Autodesk Fusion 360 part; units mm, degrees
(part 2 of 6)
sketch "Cell axial cylinder sketch (2)" plane through (0, 9.2, 0) normal (0, 1, 0) x (1, 0, 0) in component "Battery / 18650 cell B - owner-rated 3400 mAh"
  circle A0 centre (34.2, -26.95) radius 9.1
  dimension "d462" = 34.2
  dimension "d463" = 26.95
  dimension "d464" = 9.1
  measures "d462" horizontal distance of origin A0.centre
  measures "d463" vertical distance of origin A0.centre
  measures "d464" radius of A0
extrude "Blue 18650 reference cylinder'" add sketch "Cell axial cylinder sketch (2)" along normal blind 69 separate body makes body 19 in component "Battery / 18650 cell B - owner-rated 3400 mAh"
ref_plane "WorkPlane1" through (0, 0, 43) normal (0, 0, 1) x (1, 0, 0) in component "Battery / red RCY disconnect body - provisional reference"
sketch "Red battery disconnect reference body sketch" plane through (0, 0, 43) normal (0, 0, 1) x (1, 0, 0) in component "Battery / red RCY disconnect body - provisional reference"
  line L0 (29, 70) -> (41, 70)
  line L1 (41, 70) -> (41, 80)
  line L2 (41, 80) -> (29, 80)
  line L3 (29, 80) -> (29, 70)
  dimension "d469" = 29
  dimension "d470" = 70
  dimension "d471" = 12
  dimension "d472" = 10
  constraint horizontal L0
  constraint vertical L1
  constraint horizontal L2
  constraint vertical L3
  measures "d469" horizontal distance of origin L0.start
  measures "d470" vertical distance of origin L0.start
  measures "d471" horizontal distance of L0.start L0.end
  measures "d472" vertical distance of L0.end L1.end
extrude "Red battery disconnect reference body" add sketch "Red battery disconnect reference body sketch" along normal blind 4 separate body makes body 20 in component "Battery / red RCY disconnect body - provisional reference"
ref_plane "WorkPlane2" through (0, 0, 42.9) normal (0, 0, 1) x (1, 0, 0) in component "Battery / red RCY disconnect body - provisional reference"
sketch "Illustrative disconnect key groove sketch" plane through (0, 0, 42.9) normal (0, 0, 1) x (1, 0, 0) in component "Battery / red RCY disconnect body - provisional reference"
  line L0 (34.4, 69.9) -> (35.6, 69.9)
  line L1 (35.6, 69.9) -> (35.6, 80.1)
  line L2 (35.6, 80.1) -> (34.4, 80.1)
  line L3 (34.4, 80.1) -> (34.4, 69.9)
  dimension "d477" = 34.4
  dimension "d478" = 69.9
  dimension "d479" = 1.2
  dimension "d480" = 10.2
  constraint horizontal L0
  constraint vertical L1
  constraint horizontal L2
  constraint vertical L3
  measures "d477" horizontal distance of origin L0.start
  measures "d478" vertical distance of origin L0.start
  measures "d479" horizontal distance of L0.start L0.end
  measures "d480" vertical distance of L0.end L1.end
extrude "Illustrative disconnect key groove" cut sketch "Illustrative disconnect key groove sketch" along normal blind 0.7 bodies 20 in component "Battery / red RCY disconnect body - provisional reference"
ref_plane "WorkPlane1" through (0, 0, 47) normal (0, 0, 1) x (1, 0, 0) in component "Battery / red RCY disconnect mate - provisional reference"
sketch "Red battery disconnect mating reference sketch" plane through (0, 0, 47) normal (0, 0, 1) x (1, 0, 0) in component "Battery / red RCY disconnect mate - provisional reference"
  line L0 (29, 70) -> (41, 70)
  line L1 (41, 70) -> (41, 80)
  line L2 (41, 80) -> (29, 80)
  line L3 (29, 80) -> (29, 70)
  dimension "d485" = 29
  dimension "d486" = 70
  dimension "d487" = 12
  dimension "d488" = 10
  constraint horizontal L0
  constraint vertical L1
  constraint horizontal L2
  constraint vertical L3
  measures "d485" horizontal distance of origin L0.start
  measures "d486" vertical distance of origin L0.start
  measures "d487" horizontal distance of L0.start L0.end
  measures "d488" vertical distance of L0.end L1.end
extrude "Red battery disconnect mating reference" add sketch "Red battery disconnect mating reference sketch" along normal blind 2.2 separate body makes body 21 in component "Battery / red RCY disconnect mate - provisional reference"
ref_plane "WorkPlane16" through (0, 0, 37.65) normal (0, 0, 1) x (1, 0, 0) in component "01 Tapered printed housing"
sketch "Carrier bottom wall bracket sketch" plane through (0, 0, 37.65) normal (0, 0, 1) x (1, 0, 0) in component "01 Tapered printed housing"
  line L0 (36.2, 2.1) -> (43.8, 2.1)
  line L1 (43.8, 2.1) -> (43.8, 14.1)
  line L2 (43.8, 14.1) -> (36.2, 14.1)
  line L3 (36.2, 14.1) -> (36.2, 2.1)
  dimension "d493" = 36.2
  dimension "d494" = 2.1
  dimension "d495" = 7.6
  dimension "d496" = 12
  constraint horizontal L0
  constraint vertical L1
  constraint horizontal L2
  constraint vertical L3
  measures "d493" horizontal distance of origin L0.start
  measures "d494" vertical distance of origin L0.start
  measures "d495" horizontal distance of L0.start L0.end
  measures "d496" vertical distance of L0.end L1.end
extrude "Carrier bottom wall bracket" add sketch "Carrier bottom wall bracket sketch" along normal blind 6 bodies 1 in component "01 Tapered printed housing"
ref_plane "WorkPlane17" through (0, 0, 37.65) normal (0, 0, 1) x (1, 0, 0) in component "01 Tapered printed housing"
sketch "Carrier M2 boss sketch" plane through (0, 0, 37.65) normal (0, 0, 1) x (1, 0, 0) in component "01 Tapered printed housing"
  circle A0 centre (6, 18) radius 3.8
  dimension "d501" = 6
  dimension "d502" = 18
  dimension "d503" = 3.8
  measures "d501" horizontal distance of origin A0.centre
  measures "d502" vertical distance of origin A0.centre
  measures "d503" radius of A0
extrude "Carrier M2 boss" add sketch "Carrier M2 boss sketch" along normal blind 6 bodies 1 in component "01 Tapered printed housing"
ref_plane "WorkPlane18" through (0, 0, 39.65) normal (0, 0, 1) x (1, 0, 0) in component "01 Tapered printed housing"
sketch "Carrier insert pocket sketch" plane through (0, 0, 39.65) normal (0, 0, 1) x (1, 0, 0) in component "01 Tapered printed housing"
  circle A0 centre (6, 18) radius 1.65
  dimension "d508" = 6
  dimension "d509" = 18
  dimension "d510" = 1.65
  measures "d508" horizontal distance of origin A0.centre
  measures "d509" vertical distance of origin A0.centre
  measures "d510" radius of A0
extrude "Carrier insert pocket" cut sketch "Carrier insert pocket sketch" along normal blind 4.1 bodies 1 in component "01 Tapered printed housing"
ref_plane "WorkPlane19" through (0, 0, 37.65) normal (0, 0, 1) x (1, 0, 0) in component "01 Tapered printed housing"
sketch "Carrier M2 boss sketch (1)" plane through (0, 0, 37.65) normal (0, 0, 1) x (1, 0, 0) in component "01 Tapered printed housing"
  circle A0 centre (6, 77) radius 3.8
  dimension "d515" = 6
  dimension "d516" = 77
  dimension "d517" = 3.8
  measures "d515" horizontal distance of origin A0.centre
  measures "d516" vertical distance of origin A0.centre
  measures "d517" radius of A0
extrude "Carrier M2 boss (1)" add sketch "Carrier M2 boss sketch (1)" along normal blind 6 bodies 1 in component "01 Tapered printed housing"
ref_plane "WorkPlane20" through (0, 0, 39.65) normal (0, 0, 1) x (1, 0, 0) in component "01 Tapered printed housing"
sketch "Carrier insert pocket sketch (1)" plane through (0, 0, 39.65) normal (0, 0, 1) x (1, 0, 0) in component "01 Tapered printed housing"
  circle A0 centre (6, 77) radius 1.65
  dimension "d522" = 6
  dimension "d523" = 77
  dimension "d524" = 1.65
  measures "d522" horizontal distance of origin A0.centre
  measures "d523" vertical distance of origin A0.centre
  measures "d524" radius of A0
extrude "Carrier insert pocket (1)" cut sketch "Carrier insert pocket sketch (1)" along normal blind 4.1 bodies 1 in component "01 Tapered printed housing"
ref_plane "WorkPlane21" through (0, 0, 37.65) normal (0, 0, 1) x (1, 0, 0) in component "01 Tapered printed housing"
sketch "Carrier M2 boss sketch (2)" plane through (0, 0, 37.65) normal (0, 0, 1) x (1, 0, 0) in component "01 Tapered printed housing"
  circle A0 centre (40, 14) radius 3.8
  dimension "d529" = 40
  dimension "d530" = 14
  dimension "d531" = 3.8
  measures "d529" horizontal distance of origin A0.centre
  measures "d530" vertical distance of origin A0.centre
  measures "d531" radius of A0
extrude "Carrier M2 boss (2)" add sketch "Carrier M2 boss sketch (2)" along normal blind 6 bodies 1 in component "01 Tapered printed housing"
ref_plane "WorkPlane22" through (0, 0, 39.65) normal (0, 0, 1) x (1, 0, 0) in component "01 Tapered printed housing"
sketch "Carrier insert pocket sketch (2)" plane through (0, 0, 39.65) normal (0, 0, 1) x (1, 0, 0) in component "01 Tapered printed housing"
  circle A0 centre (40, 14) radius 1.65
  dimension "d536" = 40
  dimension "d537" = 14
  dimension "d538" = 1.65
  measures "d536" horizontal distance of origin A0.centre
  measures "d537" vertical distance of origin A0.centre
  measures "d538" radius of A0
extrude "Carrier insert pocket (2)" cut sketch "Carrier insert pocket sketch (2)" along normal blind 4.1 bodies 1 in component "01 Tapered printed housing"
ref_plane "WorkPlane1" through (0, 0, 43.65) normal (0, 0, 1) x (1, 0, 0) in component "Carrier / removable electronics plate"
sketch "Shaped electronics carrier sketch" plane through (0, 0, 43.65) normal (0, 0, 1) x (1, 0, 0) in component "Carrier / removable electronics plate"
  line L0 (2.7, 10.4) -> (43.6, 10.4)
  line L1 (43.6, 10.4) -> (43.6, 83.6)
  line L2 (43.6, 83.6) -> (2.7, 83.6)
  line L3 (2.7, 83.6) -> (2.7, 10.4)
  dimension "d543" = 2.7
  dimension "d544" = 10.4
  dimension "d545" = 40.9
  dimension "d546" = 73.2
  constraint horizontal L0
  constraint vertical L1
  constraint horizontal L2
  constraint vertical L3
  measures "d543" horizontal distance of origin L0.start
  measures "d544" vertical distance of origin L0.start
  measures "d545" horizontal distance of L0.start L0.end
  measures "d546" vertical distance of L0.end L1.end
extrude "Shaped electronics carrier" add sketch "Shaped electronics carrier sketch" along normal blind 2 separate body makes body 22 in component "Carrier / removable electronics plate"
ref_plane "WorkPlane1" through (0, 0, 45.65) normal (0, 0, 1) x (1, 0, 0) in component "Carrier / future PCB allocation — layout pending"
sketch "Reshaped future PCB sketch" plane through (0, 0, 45.65) normal (0, 0, 1) x (1, 0, 0) in component "Carrier / future PCB allocation — layout pending"
  line L0 (3.6, 12) -> (43, 12)
  line L1 (43, 12) -> (43, 82.4)
  line L2 (43, 82.4) -> (3.6, 82.4)
  line L3 (3.6, 82.4) -> (3.6, 12)
  dimension "d551" = 3.6
  dimension "d552" = 12
  dimension "d553" = 39.4
  dimension "d554" = 70.4
  constraint horizontal L0
  constraint vertical L1
  constraint horizontal L2
  constraint vertical L3
  measures "d551" horizontal distance of origin L0.start
  measures "d552" vertical distance of origin L0.start
  measures "d553" horizontal distance of L0.start L0.end
  measures "d554" vertical distance of L0.end L1.end
extrude "Reshaped future PCB" add sketch "Reshaped future PCB sketch" along normal blind 1.6 separate body makes body 23 in component "Carrier / future PCB allocation — layout pending"
ref_plane "WorkPlane2" through (0, 0, 43.5) normal (0, 0, 1) x (1, 0, 0) in component "Carrier / removable electronics plate"
sketch "Right button and terminal service notch sketch" plane through (0, 0, 43.5) normal (0, 0, 1) x (1, 0, 0) in component "Carrier / removable electronics plate"
  line L0 (2, 37) -> (26, 37)
  line L1 (26, 37) -> (26, 53)
  line L2 (26, 53) -> (2, 53)
  line L3 (2, 53) -> (2, 37)
  dimension "d559" = 2
  dimension "d560" = 37
  dimension "d561" = 24
  dimension "d562" = 16
  constraint horizontal L0
  constraint vertical L1
  constraint horizontal L2
  constraint vertical L3
  measures "d559" horizontal distance of origin L0.start
  measures "d560" vertical distance of origin L0.start
  measures "d561" horizontal distance of L0.start L0.end
  measures "d562" vertical distance of L0.end L1.end
extrude "Right button and terminal service notch" cut sketch "Right button and terminal service notch sketch" along normal blind 4 bodies 22 in component "Carrier / removable electronics plate"
ref_plane "WorkPlane3" through (0, 0, 43.5) normal (0, 0, 1) x (1, 0, 0) in component "Carrier / removable electronics plate"
sketch "Battery disconnect access notch sketch" plane through (0, 0, 43.5) normal (0, 0, 1) x (1, 0, 0) in component "Carrier / removable electronics plate"
  line L0 (28, 67) -> (44, 67)
  line L1 (44, 67) -> (44, 84)
  line L2 (44, 84) -> (28, 84)
  line L3 (28, 84) -> (28, 67)
  dimension "d567" = 28
  dimension "d568" = 67
  dimension "d569" = 16
  dimension "d570" = 17
  constraint horizontal L0
  constraint vertical L1
  constraint horizontal L2
  constraint vertical L3
  measures "d567" horizontal distance of origin L0.start
  measures "d568" vertical distance of origin L0.start
  measures "d569" horizontal distance of L0.start L0.end
  measures "d570" vertical distance of L0.end L1.end
extrude "Battery disconnect access notch" cut sketch "Battery disconnect access notch sketch" along normal blind 4 bodies 22 in component "Carrier / removable electronics plate"
ref_plane "WorkPlane4" through (0, 0, 43.5) normal (0, 0, 1) x (1, 0, 0) in component "Carrier / removable electronics plate"
sketch "Shared M2 mounting clearance sketch" plane through (0, 0, 43.5) normal (0, 0, 1) x (1, 0, 0) in component "Carrier / removable electronics plate"
  circle A0 centre (6, 18) radius 1.2
  dimension "d575" = 6
  dimension "d576" = 18
  dimension "d577" = 1.2
  measures "d575" horizontal distance of origin A0.centre
  measures "d576" vertical distance of origin A0.centre
  measures "d577" radius of A0
extrude "Shared M2 mounting clearance" cut sketch "Shared M2 mounting clearance sketch" along normal blind 4 bodies 22 in component "Carrier / removable electronics plate"
ref_plane "WorkPlane5" through (0, 0, 43.5) normal (0, 0, 1) x (1, 0, 0) in component "Carrier / removable electronics plate"
sketch "Shared M2 mounting clearance sketch (1)" plane through (0, 0, 43.5) normal (0, 0, 1) x (1, 0, 0) in component "Carrier / removable electronics plate"
  circle A0 centre (6, 77) radius 1.2
  dimension "d582" = 6
  dimension "d583" = 77
  dimension "d584" = 1.2
  measures "d582" horizontal distance of origin A0.centre
  measures "d583" vertical distance of origin A0.centre
  measures "d584" radius of A0
extrude "Shared M2 mounting clearance (1)" cut sketch "Shared M2 mounting clearance sketch (1)" along normal blind 4 bodies 22 in component "Carrier / removable electronics plate"
ref_plane "WorkPlane6" through (0, 0, 43.5) normal (0, 0, 1) x (1, 0, 0) in component "Carrier / removable electronics plate"
sketch "Shared M2 mounting clearance sketch (2)" plane through (0, 0, 43.5) normal (0, 0, 1) x (1, 0, 0) in component "Carrier / removable electronics plate"
  circle A0 centre (40, 14) radius 1.2
  dimension "d589" = 40
  dimension "d590" = 14
  dimension "d591" = 1.2
  measures "d589" horizontal distance of origin A0.centre
  measures "d590" vertical distance of origin A0.centre
  measures "d591" radius of A0
extrude "Shared M2 mounting clearance (2)" cut sketch "Shared M2 mounting clearance sketch (2)" along normal blind 4 bodies 22 in component "Carrier / removable electronics plate"
ref_plane "WorkPlane2" through (0, 0, 43.5) normal (0, 0, 1) x (1, 0, 0) in component "Carrier / future PCB allocation — layout pending"
sketch "Right button and terminal service notch sketch (2)" plane through (0, 0, 43.5) normal (0, 0, 1) x (1, 0, 0) in component "Carrier / future PCB allocation — layout pending"
  line L0 (2, 37) -> (26, 37)
  line L1 (26, 37) -> (26, 53)
  line L2 (26, 53) -> (2, 53)
  line L3 (2, 53) -> (2, 37)
  dimension "d596" = 2
  dimension "d597" = 37
  dimension "d598" = 24
  dimension "d599" = 16
  constraint horizontal L0
  constraint vertical L1
  constraint horizontal L2
  constraint vertical L3
  measures "d596" horizontal distance of origin L0.start
  measures "d597" vertical distance of origin L0.start
  measures "d598" horizontal distance of L0.start L0.end
  measures "d599" vertical distance of L0.end L1.end
extrude "Right button and terminal service notch'" cut sketch "Right button and terminal service notch sketch (2)" along normal blind 4 bodies 23 in component "Carrier / future PCB allocation — layout pending"
ref_plane "WorkPlane3" through (0, 0, 43.5) normal (0, 0, 1) x (1, 0, 0) in component "Carrier / future PCB allocation — layout pending"
sketch "Battery disconnect access notch sketch (2)" plane through (0, 0, 43.5) normal (0, 0, 1) x (1, 0, 0) in component "Carrier / future PCB allocation — layout pending"
  line L0 (28, 67) -> (44, 67)
  line L1 (44, 67) -> (44, 84)
  line L2 (44, 84) -> (28, 84)
  line L3 (28, 84) -> (28, 67)
  dimension "d604" = 28
  dimension "d605" = 67
  dimension "d606" = 16
  dimension "d607" = 17
  constraint horizontal L0
  constraint vertical L1
  constraint horizontal L2
  constraint vertical L3
  measures "d604" horizontal distance of origin L0.start
  measures "d605" vertical distance of origin L0.start
  measures "d606" horizontal distance of L0.start L0.end
  measures "d607" vertical distance of L0.end L1.end
extrude "Battery disconnect access notch'" cut sketch "Battery disconnect access notch sketch (2)" along normal blind 4 bodies 23 in component "Carrier / future PCB allocation — layout pending"
ref_plane "WorkPlane4" through (0, 0, 43.5) normal (0, 0, 1) x (1, 0, 0) in component "Carrier / future PCB allocation — layout pending"
sketch "Shared M2 mounting clearance sketch (3)" plane through (0, 0, 43.5) normal (0, 0, 1) x (1, 0, 0) in component "Carrier / future PCB allocation — layout pending"
  circle A0 centre (6, 18) radius 1.2
  dimension "d612" = 6
  dimension "d613" = 18
  dimension "d614" = 1.2
  measures "d612" horizontal distance of origin A0.centre
  measures "d613" vertical distance of origin A0.centre
  measures "d614" radius of A0
extrude "Shared M2 mounting clearance'" cut sketch "Shared M2 mounting clearance sketch (3)" along normal blind 4 bodies 23 in component "Carrier / future PCB allocation — layout pending"
ref_plane "WorkPlane5" through (0, 0, 43.5) normal (0, 0, 1) x (1, 0, 0) in component "Carrier / future PCB allocation — layout pending"
sketch "Shared M2 mounting clearance sketch (1) (2)" plane through (0, 0, 43.5) normal (0, 0, 1) x (1, 0, 0) in component "Carrier / future PCB allocation — layout pending"
  circle A0 centre (6, 77) radius 1.2
  dimension "d619" = 6
  dimension "d620" = 77
  dimension "d621" = 1.2
  measures "d619" horizontal distance of origin A0.centre
  measures "d620" vertical distance of origin A0.centre
  measures "d621" radius of A0
extrude "Shared M2 mounting clearance (1)'" cut sketch "Shared M2 mounting clearance sketch (1) (2)" along normal blind 4 bodies 23 in component "Carrier / future PCB allocation — layout pending"
ref_plane "WorkPlane6" through (0, 0, 43.5) normal (0, 0, 1) x (1, 0, 0) in component "Carrier / future PCB allocation — layout pending"
sketch "Shared M2 mounting clearance sketch (2) (2)" plane through (0, 0, 43.5) normal (0, 0, 1) x (1, 0, 0) in component "Carrier / future PCB allocation — layout pending"
  circle A0 centre (40, 14) radius 1.2
  dimension "d626" = 40
  dimension "d627" = 14
  dimension "d628" = 1.2
  measures "d626" horizontal distance of origin A0.centre
  measures "d627" vertical distance of origin A0.centre
  measures "d628" radius of A0
extrude "Shared M2 mounting clearance (2)'" cut sketch "Shared M2 mounting clearance sketch (2) (2)" along normal blind 4 bodies 23 in component "Carrier / future PCB allocation — layout pending"
ref_plane "WorkPlane7" through (0, 0, 47.25) normal (0, 0, 1) x (1, 0, 0) in component "Carrier / future PCB allocation — layout pending"
sketch "Power-stage allocation sketch" plane through (0, 0, 47.25) normal (0, 0, 1) x (1, 0, 0) in component "Carrier / future PCB allocation — layout pending"
  line L0 (12, 18) -> (32, 18)
  line L1 (32, 18) -> (32, 31)
  line L2 (32, 31) -> (12, 31)
  line L3 (12, 31) -> (12, 18)
  dimension "d633" = 12
  dimension "d634" = 18
  dimension "d635" = 20
  dimension "d636" = 13
  constraint horizontal L0
  constraint vertical L1
  constraint horizontal L2
  constraint vertical L3
  measures "d633" horizontal distance of origin L0.start
  measures "d634" vertical distance of origin L0.start
  measures "d635" horizontal distance of L0.start L0.end
  measures "d636" vertical distance of L0.end L1.end
extrude "Power-stage allocation" add sketch "Power-stage allocation sketch" along normal blind 3.5 separate body makes body 24 in component "Carrier / future PCB allocation — layout pending"
ref_plane "WorkPlane8" through (0, 0, 47.25) normal (0, 0, 1) x (1, 0, 0) in component "Carrier / future PCB allocation — layout pending"
sketch "Analog allocation sketch" plane through (0, 0, 47.25) normal (0, 0, 1) x (1, 0, 0) in component "Carrier / future PCB allocation — layout pending"
  line L0 (28, 40) -> (40, 40)
  line L1 (40, 40) -> (40, 59)
  line L2 (40, 59) -> (28, 59)
  line L3 (28, 59) -> (28, 40)
  dimension "d641" = 28
  dimension "d642" = 40
  dimension "d643" = 12
  dimension "d644" = 19
  constraint horizontal L0
  constraint vertical L1
  constraint horizontal L2
  constraint vertical L3
  measures "d641" horizontal distance of origin L0.start
  measures "d642" vertical distance of origin L0.start
  measures "d643" horizontal distance of L0.start L0.end
  measures "d644" vertical distance of L0.end L1.end
extrude "Analog allocation" add sketch "Analog allocation sketch" along normal blind 2.5 separate body makes body 25 in component "Carrier / future PCB allocation — layout pending"
ref_plane "WorkPlane9" through (0, 0, 47.25) normal (0, 0, 1) x (1, 0, 0) in component "Carrier / future PCB allocation — layout pending"
sketch "Digital allocation sketch" plane through (0, 0, 47.25) normal (0, 0, 1) x (1, 0, 0) in component "Carrier / future PCB allocation — layout pending"
  line L0 (12, 57) -> (24, 57)
  line L1 (24, 57) -> (24, 65)
  line L2 (24, 65) -> (12, 65)
  line L3 (12, 65) -> (12, 57)
  dimension "d649" = 12
  dimension "d650" = 57
  dimension "d651" = 12
  dimension "d652" = 8
  constraint horizontal L0
  constraint vertical L1
  constraint horizontal L2
  constraint vertical L3
  measures "d649" horizontal distance of origin L0.start
  measures "d650" vertical distance of origin L0.start
  measures "d651" horizontal distance of L0.start L0.end
  measures "d652" vertical distance of L0.end L1.end
extrude "Digital allocation" add sketch "Digital allocation sketch" along normal blind 2 separate body makes body 26 in component "Carrier / future PCB allocation — layout pending"
ref_plane "WorkPlane1" through (0, 0, -7) normal (0, 0, 1) x (1, 0, 0) in component "M2 x 7 socket_cap screw — GEN-M2-SHCS-L7-AF1.5"
sketch "Joined screw sketch (2)" plane through (0, 0, -7) normal (0, 0, 1) x (1, 0, 0) in component "M2 x 7 socket_cap screw — GEN-M2-SHCS-L7-AF1.5"
  circle A0 centre (0, 0) radius 0.95
  dimension "d657" = 0.95
  measures "d657" radius of A0
extrude "Joined screw'" add sketch "Joined screw sketch (2)" along normal blind 7 separate body makes body 27 in component "M2 x 7 socket_cap screw — GEN-M2-SHCS-L7-AF1.5"
ref_plane "WorkPlane2" through (0, 0, 0) normal (0, 0, 1) x (1, 0, 0) in component "M2 x 7 socket_cap screw — GEN-M2-SHCS-L7-AF1.5"
sketch "Screw head sketch (2)" plane through (0, 0, 0) normal (0, 0, 1) x (1, 0, 0) in component "M2 x 7 socket_cap screw — GEN-M2-SHCS-L7-AF1.5"
  circle A0 centre (0, 0) radius 1.9
  dimension "d662" = 1.9
  measures "d662" radius of A0
extrude "Screw head'" add sketch "Screw head sketch (2)" along normal blind 2 bodies 27 in component "M2 x 7 socket_cap screw — GEN-M2-SHCS-L7-AF1.5"
fillet "Rounded head crown'" radius 0.15 1 edges at (-1.7714, -0.6871, 2) on bodies 27 in component "M2 x 7 socket_cap screw — GEN-M2-SHCS-L7-AF1.5"
ref_plane "WorkPlane3" through (0, 0, 1) normal (0, 0, 1) x (1, 0, 0) in component "M2 x 7 socket_cap screw — GEN-M2-SHCS-L7-AF1.5"
sketch "Hex drive 1.5 mm across flats" plane through (0, 0, 1) normal (0, 0, 1) x (1, 0, 0) in component "M2 x 7 socket_cap screw — GEN-M2-SHCS-L7-AF1.5"
  line L0 (0.866, 0) -> (0.433, 0.75)
  line L1 (0.433, 0.75) -> (-0.433, 0.75)
  line L2 (-0.433, 0.75) -> (-0.866, 0)
  line L3 (-0.866, 0) -> (-0.433, -0.75)
  line L4 (-0.433, -0.75) -> (0.433, -0.75)
  line L5 (0.433, -0.75) -> (0.866, 0)
extrude "Hex drive recess'" cut sketch "Hex drive 1.5 mm across flats" along normal blind 1.1 bodies 27 in component "M2 x 7 socket_cap screw — GEN-M2-SHCS-L7-AF1.5"
ref_plane "WorkPlane1" through (0, 0, -4) normal (0, 0, 1) x (1, 0, 0) in component "M2 insert OD3.2 x 4 — GEN-M2-HEATSET-OD3.2-L4"
sketch "Hollow insert sketch (2)" plane through (0, 0, -4) normal (0, 0, 1) x (1, 0, 0) in component "M2 insert OD3.2 x 4 — GEN-M2-HEATSET-OD3.2-L4"
  circle A0 centre (0, 0) radius 1.6
  dimension "d673" = 1.6
  measures "d673" radius of A0
extrude "Hollow insert'" add sketch "Hollow insert sketch (2)" along normal blind 4 separate body makes body 28 in component "M2 insert OD3.2 x 4 — GEN-M2-HEATSET-OD3.2-L4"
ref_plane "WorkPlane2" through (0, 0, -4.1) normal (0, 0, 1) x (1, 0, 0) in component "M2 insert OD3.2 x 4 — GEN-M2-HEATSET-OD3.2-L4"
sketch "Unthreaded insert bore sketch (2)" plane through (0, 0, -4.1) normal (0, 0, 1) x (1, 0, 0) in component "M2 insert OD3.2 x 4 — GEN-M2-HEATSET-OD3.2-L4"
  circle A0 centre (0, 0) radius 1.05
  dimension "d678" = 1.05
  measures "d678" radius of A0
extrude "Unthreaded insert bore'" cut sketch "Unthreaded insert bore sketch (2)" along normal blind 4.2 bodies 28 in component "M2 insert OD3.2 x 4 — GEN-M2-HEATSET-OD3.2-L4"
ref_plane "WorkPlane3" through (0, 0, -3) normal (0, 0, 1) x (1, 0, 0) in component "M2 insert OD3.2 x 4 — GEN-M2-HEATSET-OD3.2-L4"
sketch "Cosmetic insert relief (2)" plane through (0, 0, -3) normal (0, 0, 1) x (1, 0, 0) in component "M2 insert OD3.2 x 4 — GEN-M2-HEATSET-OD3.2-L4"
  circle A0 centre (0, 0) radius 1.7
  circle A1 centre (0, 0) radius 1.5
  dimension "d683" = 1.7
  dimension "d684" = 1.5
  measures "d683" radius of A0
  measures "d684" radius of A1
extrude "Cosmetic annular relief'" cut sketch "Cosmetic insert relief (2)" along normal blind 0.25 bodies 28 in component "M2 insert OD3.2 x 4 — GEN-M2-HEATSET-OD3.2-L4"
ref_plane "WorkPlane4" through (0, 0, -1) normal (0, 0, 1) x (1, 0, 0) in component "M2 insert OD3.2 x 4 — GEN-M2-HEATSET-OD3.2-L4"
sketch "Cosmetic insert relief (1) (2)" plane through (0, 0, -1) normal (0, 0, 1) x (1, 0, 0) in component "M2 insert OD3.2 x 4 — GEN-M2-HEATSET-OD3.2-L4"
  circle A0 centre (0, 0) radius 1.7
  circle A1 centre (0, 0) radius 1.5
  dimension "d689" = 1.7
  dimension "d690" = 1.5
  measures "d689" radius of A0
  measures "d690" radius of A1
extrude "Cosmetic annular relief (1)'" cut sketch "Cosmetic insert relief (1) (2)" along normal blind 0.25 bodies 28 in component "M2 insert OD3.2 x 4 — GEN-M2-HEATSET-OD3.2-L4"
ref_plane "WorkPlane23" through (0, 0, 14.3) normal (0, 0, 1) x (1, 0, 0) in component "01 Tapered printed housing"
sketch "Lower display retainer wall bracket sketch" plane through (0, 0, 14.3) normal (0, 0, 1) x (1, 0, 0) in component "01 Tapered printed housing"
  line L0 (48.2, 2.1) -> (55.8, 2.1)
  line L1 (55.8, 2.1) -> (55.8, 11.1)
  line L2 (55.8, 11.1) -> (48.2, 11.1)
  line L3 (48.2, 11.1) -> (48.2, 2.1)
  dimension "d695" = 48.2
  dimension "d696" = 2.1
  dimension "d697" = 7.6
  dimension "d698" = 9
  constraint horizontal L0
  constraint vertical L1
  constraint horizontal L2
  constraint vertical L3
  measures "d695" horizontal distance of origin L0.start
  measures "d696" vertical distance of origin L0.start
  measures "d697" horizontal distance of L0.start L0.end
  measures "d698" vertical distance of L0.end L1.end
extrude "Lower display retainer wall bracket" add sketch "Lower display retainer wall bracket sketch" along normal blind 6 bodies 1 in component "01 Tapered printed housing"
ref_plane "WorkPlane24" through (0, 0, 14.3) normal (0, 0, 1) x (1, 0, 0) in component "01 Tapered printed housing"
sketch "Display retainer M2 boss sketch" plane through (0, 0, 14.3) normal (0, 0, 1) x (1, 0, 0) in component "01 Tapered printed housing"
  circle A0 centre (52, 11) radius 3.8
  dimension "d703" = 52
  dimension "d704" = 11
  dimension "d705" = 3.8
  measures "d703" horizontal distance of origin A0.centre
  measures "d704" vertical distance of origin A0.centre
  measures "d705" radius of A0
extrude "Display retainer M2 boss" add sketch "Display retainer M2 boss sketch" along normal blind 6 bodies 1 in component "01 Tapered printed housing"
ref_plane "WorkPlane25" through (0, 0, 16.3) normal (0, 0, 1) x (1, 0, 0) in component "01 Tapered printed housing"
sketch "Display retainer insert pocket sketch" plane through (0, 0, 16.3) normal (0, 0, 1) x (1, 0, 0) in component "01 Tapered printed housing"
  circle A0 centre (52, 11) radius 1.65
  dimension "d710" = 52
  dimension "d711" = 11
  dimension "d712" = 1.65
  measures "d710" horizontal distance of origin A0.centre
  measures "d711" vertical distance of origin A0.centre
  measures "d712" radius of A0
extrude "Display retainer insert pocket" cut sketch "Display retainer insert pocket sketch" along normal blind 4.1 bodies 1 in component "01 Tapered printed housing"
ref_plane "WorkPlane26" through (0, 0, 14.3) normal (0, 0, 1) x (1, 0, 0) in component "01 Tapered printed housing"
sketch "Display retainer M2 boss sketch (1)" plane through (0, 0, 14.3) normal (0, 0, 1) x (1, 0, 0) in component "01 Tapered printed housing"
  circle A0 centre (14, 119) radius 3.8
  dimension "d717" = 14
  dimension "d718" = 119
  dimension "d719" = 3.8
  measures "d717" horizontal distance of origin A0.centre
  measures "d718" vertical distance of origin A0.centre
  measures "d719" radius of A0
extrude "Display retainer M2 boss (1)" add sketch "Display retainer M2 boss sketch (1)" along normal blind 6 bodies 1 in component "01 Tapered printed housing"
ref_plane "WorkPlane27" through (0, 0, 16.3) normal (0, 0, 1) x (1, 0, 0) in component "01 Tapered printed housing"
sketch "Display retainer insert pocket sketch (1)" plane through (0, 0, 16.3) normal (0, 0, 1) x (1, 0, 0) in component "01 Tapered printed housing"
  circle A0 centre (14, 119) radius 1.65
  dimension "d724" = 14
  dimension "d725" = 119
  dimension "d726" = 1.65
  measures "d724" horizontal distance of origin A0.centre
  measures "d725" vertical distance of origin A0.centre
  measures "d726" radius of A0
extrude "Display retainer insert pocket (1)" cut sketch "Display retainer insert pocket sketch (1)" along normal blind 4.1 bodies 1 in component "01 Tapered printed housing"
ref_plane "WorkPlane1" through (0, 0, 20.3) normal (0, 0, 1) x (1, 0, 0) in component "Display / lower removable retainer concept"
sketch "lower clip screw seat sketch" plane through (0, 0, 20.3) normal (0, 0, 1) x (1, 0, 0) in component "Display / lower removable retainer concept"
  line L0 (48.6, 7.5) -> (60, 7.5)
  line L1 (60, 7.5) -> (60, 14.5)
  line L2 (60, 14.5) -> (48.6, 14.5)
  line L3 (48.6, 14.5) -> (48.6, 7.5)
  dimension "d731" = 48.6
  dimension "d732" = 7.5
  dimension "d733" = 11.4
  dimension "d734" = 7
  constraint horizontal L0
  constraint vertical L1
  constraint horizontal L2
  constraint vertical L3
  measures "d731" horizontal distance of origin L0.start
  measures "d732" vertical distance of origin L0.start
  measures "d733" horizontal distance of L0.start L0.end
  measures "d734" vertical distance of L0.end L1.end
extrude "lower clip screw seat" add sketch "lower clip screw seat sketch" along normal blind 2 separate body makes body 29 in component "Display / lower removable retainer concept"
ref_plane "WorkPlane2" through (0, 0, 14.2) normal (0, 0, 1) x (1, 0, 0) in component "Display / lower removable retainer concept"
sketch "Flat frame contact provision sketch" plane through (0, 0, 14.2) normal (0, 0, 1) x (1, 0, 0) in component "Display / lower removable retainer concept"
  line L0 (58, 5.5) -> (60, 5.5)
  line L1 (60, 5.5) -> (60, 9.5)
  line L2 (60, 9.5) -> (58, 9.5)
  line L3 (58, 9.5) -> (58, 5.5)
  dimension "d739" = 58
  dimension "d740" = 5.5
  dimension "d741" = 2
  dimension "d742" = 4
  constraint horizontal L0
  constraint vertical L1
  constraint horizontal L2
  constraint vertical L3
  measures "d739" horizontal distance of origin L0.start
  measures "d740" vertical distance of origin L0.start
  measures "d741" horizontal distance of L0.start L0.end
  measures "d742" vertical distance of L0.end L1.end
extrude "Flat frame contact provision" add sketch "Flat frame contact provision sketch" along normal blind 8.1 bodies 29 in component "Display / lower removable retainer concept"
ref_plane "WorkPlane3" through (0, 0, 20.2) normal (0, 0, 1) x (1, 0, 0) in component "Display / lower removable retainer concept"
sketch "M2 retainer clearance sketch" plane through (0, 0, 20.2) normal (0, 0, 1) x (1, 0, 0) in component "Display / lower removable retainer concept"
  circle A0 centre (52, 11) radius 1.2
  dimension "d747" = 52
  dimension "d748" = 11
  dimension "d749" = 1.2
  measures "d747" horizontal distance of origin A0.centre
  measures "d748" vertical distance of origin A0.centre
  measures "d749" radius of A0
extrude "M2 retainer clearance" cut sketch "M2 retainer clearance sketch" along normal blind 2.2 bodies 29 in component "Display / lower removable retainer concept"
ref_plane "WorkPlane1" through (0, 0, 20.3) normal (0, 0, 1) x (1, 0, 0) in component "Display / upper removable retainer concept"
sketch "upper clip screw seat sketch" plane through (0, 0, 20.3) normal (0, 0, 1) x (1, 0, 0) in component "Display / upper removable retainer concept"
  line L0 (8, 115.5) -> (17.4, 115.5)
  line L1 (17.4, 115.5) -> (17.4, 122.5)
  line L2 (17.4, 122.5) -> (8, 122.5)
  line L3 (8, 122.5) -> (8, 115.5)
  dimension "d754" = 8
  dimension "d755" = 115.5
  dimension "d756" = 9.4
  dimension "d757" = 7
  constraint horizontal L0
  constraint vertical L1
  constraint horizontal L2
  constraint vertical L3
  measures "d754" horizontal distance of origin L0.start
  measures "d755" vertical distance of origin L0.start
  measures "d756" horizontal distance of L0.start L0.end
  measures "d757" vertical distance of L0.end L1.end
extrude "upper clip screw seat" add sketch "upper clip screw seat sketch" along normal blind 2 separate body makes body 30 in component "Display / upper removable retainer concept"
ref_plane "WorkPlane2" through (0, 0, 14.2) normal (0, 0, 1) x (1, 0, 0) in component "Display / upper removable retainer concept"
sketch "Flat frame contact provision sketch (2)" plane through (0, 0, 14.2) normal (0, 0, 1) x (1, 0, 0) in component "Display / upper removable retainer concept"
  line L0 (8, 117) -> (10, 117)
  line L1 (10, 117) -> (10, 121)
  line L2 (10, 121) -> (8, 121)
  line L3 (8, 121) -> (8, 117)
  dimension "d762" = 8
  dimension "d763" = 117
  dimension "d764" = 2
  dimension "d765" = 4
  constraint horizontal L0
  constraint vertical L1
  constraint horizontal L2
  constraint vertical L3
  measures "d762" horizontal distance of origin L0.start
  measures "d763" vertical distance of origin L0.start
  measures "d764" horizontal distance of L0.start L0.end
  measures "d765" vertical distance of L0.end L1.end
extrude "Flat frame contact provision'" add sketch "Flat frame contact provision sketch (2)" along normal blind 8.1 bodies 30 in component "Display / upper removable retainer concept"
ref_plane "WorkPlane3" through (0, 0, 20.2) normal (0, 0, 1) x (1, 0, 0) in component "Display / upper removable retainer concept"
sketch "M2 retainer clearance sketch (2)" plane through (0, 0, 20.2) normal (0, 0, 1) x (1, 0, 0) in component "Display / upper removable retainer concept"
  circle A0 centre (14, 119) radius 1.2
  dimension "d770" = 14
  dimension "d771" = 119
  dimension "d772" = 1.2
  measures "d770" horizontal distance of origin A0.centre
  measures "d771" vertical distance of origin A0.centre
  measures "d772" radius of A0
extrude "M2 retainer clearance'" cut sketch "M2 retainer clearance sketch (2)" along normal blind 2.2 bodies 30 in component "Display / upper removable retainer concept"
ref_plane "WorkPlane1" through (0, 0, -5) normal (0, 0, 1) x (1, 0, 0) in component "M2 x 5 socket_cap screw — GEN-M2-SHCS-L5-AF1.5"
sketch "Joined screw sketch (3)" plane through (0, 0, -5) normal (0, 0, 1) x (1, 0, 0) in component "M2 x 5 socket_cap screw — GEN-M2-SHCS-L5-AF1.5"
  circle A0 centre (0, 0) radius 0.95
  dimension "d777" = 0.95
  measures "d777" radius of A0
extrude "Joined screw''" add sketch "Joined screw sketch (3)" along normal blind 5 separate body makes body 31 in component "M2 x 5 socket_cap screw — GEN-M2-SHCS-L5-AF1.5"
ref_plane "WorkPlane2" through (0, 0, 0) normal (0, 0, 1) x (1, 0, 0) in component "M2 x 5 socket_cap screw — GEN-M2-SHCS-L5-AF1.5"
sketch "Screw head sketch (3)" plane through (0, 0, 0) normal (0, 0, 1) x (1, 0, 0) in component "M2 x 5 socket_cap screw — GEN-M2-SHCS-L5-AF1.5"
  circle A0 centre (0, 0) radius 1.9
  dimension "d782" = 1.9
  measures "d782" radius of A0
extrude "Screw head''" add sketch "Screw head sketch (3)" along normal blind 2 bodies 31 in component "M2 x 5 socket_cap screw — GEN-M2-SHCS-L5-AF1.5"
fillet "Rounded head crown''" radius 0.15 1 edges at (-1.7714, -0.6871, 2) on bodies 31 in component "M2 x 5 socket_cap screw — GEN-M2-SHCS-L5-AF1.5"
ref_plane "WorkPlane3" through (0, 0, 1) normal (0, 0, 1) x (1, 0, 0) in component "M2 x 5 socket_cap screw — GEN-M2-SHCS-L5-AF1.5"
sketch "Hex drive 1.5 mm across flats (2)" plane through (0, 0, 1) normal (0, 0, 1) x (1, 0, 0) in component "M2 x 5 socket_cap screw — GEN-M2-SHCS-L5-AF1.5"
  line L0 (0.866, 0) -> (0.433, 0.75)
  line L1 (0.433, 0.75) -> (-0.433, 0.75)
  line L2 (-0.433, 0.75) -> (-0.866, 0)
  line L3 (-0.866, 0) -> (-0.433, -0.75)
  line L4 (-0.433, -0.75) -> (0.433, -0.75)
  line L5 (0.433, -0.75) -> (0.866, 0)
extrude "Hex drive recess''" cut sketch "Hex drive 1.5 mm across flats (2)" along normal blind 1.1 bodies 31 in component "M2 x 5 socket_cap screw — GEN-M2-SHCS-L5-AF1.5"
ref_plane "WorkPlane1" through (0.15, 0, 0) normal (1, 0, 0) x (0, 1, 0) in component "Controls / right 1NO power button body"
sketch "12 mm button barrel sketch" plane through (0.15, 0, 0) normal (1, 0, 0) x (0, 0, -1) in component "Controls / right 1NO power button body"
  circle A0 centre (-44.5, 45) radius 5.8
  dimension "d794" = 45
  dimension "d795" = 5.8
  measures "d794" vertical distance of origin A0.centre
  measures "d795" radius of A0
extrude "12 mm button barrel" add sketch "12 mm button barrel sketch" along normal blind 17.85 separate body makes body 32 in component "Controls / right 1NO power button body"
ref_plane "WorkPlane2" through (-1.5, 0, 0) normal (1, 0, 0) x (0, 1, 0) in component "Controls / right 1NO power button body"
sketch "External button bezel sketch" plane through (-1.5, 0, 0) normal (1, 0, 0) x (0, 0, -1) in component "Controls / right 1NO power button body"
  circle A0 centre (-44.5, 45) radius 7
  dimension "d801" = 45
  dimension "d802" = 7
  measures "d801" vertical distance of origin A0.centre
  measures "d802" radius of A0
extrude "External button bezel" add sketch "External button bezel sketch" along normal blind 1.5 separate body makes body 33 in component "Controls / right 1NO power button body"
ref_plane "WorkPlane3" through (18, 0, 0) normal (1, 0, 0) x (0, 1, 0) in component "Controls / right 1NO power button body"
sketch "Button terminal block allowance sketch" plane through (18, 0, 0) normal (1, 0, 0) x (0, 0, -1) in component "Controls / right 1NO power button body"
  line L0 (-48.5, 41) -> (-40.5, 41)
  line L1 (-40.5, 41) -> (-40.5, 49)
  line L2 (-40.5, 49) -> (-48.5, 49)
  line L3 (-48.5, 49) -> (-48.5, 41)
  dimension "d807" = 48.5
  dimension "d808" = 41
  dimension "d809" = 8
  dimension "d810" = 8
  constraint horizontal L0
  constraint vertical L1
  constraint horizontal L2
  constraint vertical L3
  measures "d807" horizontal distance of origin L0.start
  measures "d808" vertical distance of origin L0.start
  measures "d809" horizontal distance of L0.start L0.end
  measures "d810" vertical distance of L0.end L1.end
extrude "Button terminal block allowance" add sketch "Button terminal block allowance sketch" along normal blind 7 separate body makes body 34 in component "Controls / right 1NO power button body"
ref_plane "WorkPlane1" through (-1.7, 0, 0) normal (1, 0, 0) x (0, 1, 0) in component "Controls / green momentary power cap"
sketch "Green 1NO button face sketch" plane through (-1.7, 0, 0) normal (1, 0, 0) x (0, 0, -1) in component "Controls / green momentary power cap"
  circle A0 centre (-44.5, 45) radius 4.5
  dimension "d816" = 45
  dimension "d817" = 4.5
  measures "d816" vertical distance of origin A0.centre
  measures "d817" radius of A0
extrude "Green 1NO button face" add sketch "Green 1NO button face sketch" along normal blind 0.2 separate body makes body 35 in component "Controls / green momentary power cap"
ref_plane "WorkPlane28" through (0, 0, 52.25) normal (0, 0, 1) x (1, 0, 0) in component "01 Tapered printed housing"
sketch "Rear cover bearing pad clearance sketch" plane through (0, 0, 52.25) normal (0, 0, 1) x (1, 0, 0) in component "01 Tapered printed housing"
  circle A0 centre (6, 6) radius 5.3
  dimension "d822" = 6
  dimension "d823" = 6
  dimension "d824" = 5.3
  measures "d822" horizontal distance of origin A0.centre
  measures "d823" vertical distance of origin A0.centre
  measures "d824" radius of A0
ref_plane "WorkPlane29" through (0, 0, 52.25) normal (0, 0, 1) x (1, 0, 0) in component "01 Tapered printed housing"
sketch "Rear cover bearing pad clearance sketch (1)" plane through (0, 0, 52.25) normal (0, 0, 1) x (1, 0, 0) in component "01 Tapered printed housing"
  circle A0 centre (6, 119) radius 5.3
  dimension "d829" = 6
  dimension "d830" = 119
  dimension "d831" = 5.3
  measures "d829" horizontal distance of origin A0.centre
  measures "d830" vertical distance of origin A0.centre
  measures "d831" radius of A0
ref_plane "WorkPlane30" through (0, 0, 52.25) normal (0, 0, 1) x (1, 0, 0) in component "01 Tapered printed housing"
sketch "Rear cover bearing pad clearance sketch (2)" plane through (0, 0, 52.25) normal (0, 0, 1) x (1, 0, 0) in component "01 Tapered printed housing"
  circle A0 centre (69, 6) radius 5.3
  dimension "d836" = 69
  dimension "d837" = 6
  dimension "d838" = 5.3
  measures "d836" horizontal distance of origin A0.centre
  measures "d837" vertical distance of origin A0.centre
  measures "d838" radius of A0
ref_plane "WorkPlane31" through (0, 0, 52.25) normal (0, 0, 1) x (1, 0, 0) in component "01 Tapered printed housing"
sketch "Rear cover bearing pad clearance sketch (3)" plane through (0, 0, 52.25) normal (0, 0, 1) x (1, 0, 0) in component "01 Tapered printed housing"
  circle A0 centre (69, 119) radius 5.3
  dimension "d843" = 69
  dimension "d844" = 119
  dimension "d845" = 5.3
  measures "d843" horizontal distance of origin A0.centre
  measures "d844" vertical distance of origin A0.centre
  measures "d845" radius of A0
ref_plane "WorkPlane1" through (72.6, 0, 0) normal (1, 0, 0) x (0, 1, 0) in component "USB — removable metal faceplate — local 1.80 mm seat"
sketch "Metal panel insert with 0.25 mm perimeter clearance sketch" plane through (72.6, 0, 0) normal (1, 0, 0) x (0, 0, -1) in component "USB — removable metal faceplate — local 1.80 mm seat"
  line L0 (-34.75, 6.25) -> (-19.25, 6.25)
  line L1 (-19.25, 6.25) -> (-19.25, 25.75)
  line L2 (-19.25, 25.75) -> (-34.75, 25.75)
  line L3 (-34.75, 25.75) -> (-34.75, 6.25)
  dimension "d914" = 34.75
  dimension "d915" = 6.25
  dimension "d916" = 15.5
  dimension "d917" = 19.5
  constraint horizontal L0
  constraint vertical L1
  constraint horizontal L2
  constraint vertical L3
  measures "d914" horizontal distance of origin L0.start
  measures "d915" vertical distance of origin L0.start
  measures "d916" horizontal distance of L0.start L0.end
  measures "d917" vertical distance of L0.end L1.end
extrude "Metal panel insert with 0.25 mm perimeter clearance" add sketch "Metal panel insert with 0.25 mm perimeter clearance sketch" along normal blind 2.3 separate body makes body 36 in component "USB — removable metal faceplate — local 1.80 mm seat"
ref_plane "WorkPlane1" through (70.6, 0, 0) normal (1, 0, 0) x (0, 1, 0) in component "USB — removable panel insert and board supports"
sketch "Interior printed USB backing flange sketch" plane through (70.6, 0, 0) normal (1, 0, 0) x (0, 0, -1) in component "USB — removable panel insert and board supports"
  line L0 (-37, 4) -> (-17, 4)
  line L1 (-17, 4) -> (-17, 28)
  line L2 (-17, 28) -> (-37, 28)
  line L3 (-37, 28) -> (-37, 4)
  dimension "d922" = 37
  dimension "d923" = 4
  dimension "d924" = 20
  dimension "d925" = 24
  constraint horizontal L0
  constraint vertical L1
  constraint horizontal L2
  constraint vertical L3
  measures "d922" horizontal distance of origin L0.start
  measures "d923" vertical distance of origin L0.start
  measures "d924" horizontal distance of L0.start L0.end
  measures "d925" vertical distance of L0.end L1.end
extrude "Interior printed USB backing flange" add sketch "Interior printed USB backing flange sketch" along normal blind 2 separate body makes body 37 in component "USB — removable panel insert and board supports"
ref_plane "WorkPlane2" through (70.5, 0, 0) normal (1, 0, 0) x (0, 1, 0) in component "USB — removable panel insert and board supports"
sketch "Printed frame connector interior relief sketch" plane through (70.5, 0, 0) normal (1, 0, 0) x (0, 0, -1) in component "USB — removable panel insert and board supports"
  line L0 (-30.5, 9.5) -> (-23.5, 9.5)
  line L1 (-23.5, 9.5) -> (-23.5, 22.5)
  line L2 (-23.5, 22.5) -> (-30.5, 22.5)
  line L3 (-30.5, 22.5) -> (-30.5, 9.5)
  dimension "d930" = 30.5
  dimension "d931" = 9.5
  dimension "d932" = 7
  dimension "d933" = 13
  constraint horizontal L0
  constraint vertical L1
  constraint horizontal L2
  constraint vertical L3
  measures "d930" horizontal distance of origin L0.start
  measures "d931" vertical distance of origin L0.start
  measures "d932" horizontal distance of L0.start L0.end
  measures "d933" vertical distance of L0.end L1.end
extrude "Printed frame connector interior relief" cut sketch "Printed frame connector interior relief sketch" along normal blind 2.2 bodies 37 in component "USB — removable panel insert and board supports"
ref_plane "WorkPlane2" through (72.5, 0, 0) normal (1, 0, 0) x (0, 1, 0) in component "USB — removable metal faceplate — local 1.80 mm seat"
sketch "Metal faceplate local 1.80 mm seat relief sketch" plane through (72.5, 0, 0) normal (1, 0, 0) x (0, 0, -1) in component "USB — removable metal faceplate — local 1.80 mm seat"
  line L0 (-30.5, 9.5) -> (-23.5, 9.5)
  line L1 (-23.5, 9.5) -> (-23.5, 22.5)
  line L2 (-23.5, 22.5) -> (-30.5, 22.5)
  line L3 (-30.5, 22.5) -> (-30.5, 9.5)
  dimension "d938" = 30.5
  dimension "d939" = 9.5
  dimension "d940" = 7
  dimension "d941" = 13
  constraint horizontal L0
  constraint vertical L1
  constraint horizontal L2
  constraint vertical L3
  measures "d938" horizontal distance of origin L0.start
  measures "d939" vertical distance of origin L0.start
  measures "d940" horizontal distance of L0.start L0.end
  measures "d941" vertical distance of L0.end L1.end
extrude "Metal faceplate local 1.80 mm seat relief" cut sketch "Metal faceplate local 1.80 mm seat relief sketch" along normal blind 0.6 bodies 36 in component "USB — removable metal faceplate — local 1.80 mm seat"
ref_plane "WorkPlane3" through (73.09, 0, 0) normal (1, 0, 0) x (0, 1, 0) in component "USB — removable metal faceplate — local 1.80 mm seat"
sketch "GCT 8.44 x 2.66 throat R1.05 profile" plane through (73.09, 0, 0) normal (1, 0, 0) x (0, 0, -1) in component "USB — removable metal faceplate — local 1.80 mm seat"
  line L0 (-25.67, 12.83) -> (-25.67, 19.17)
  arc A0 (-25.67, 19.17) -> (-26.72, 20.22) centre (-26.72, 19.17) ccw
  line L1 (-26.72, 20.22) -> (-27.28, 20.22)
  arc A1 (-27.28, 20.22) -> (-28.33, 19.17) centre (-27.28, 19.17) ccw
  line L2 (-28.33, 19.17) -> (-28.33, 12.83)
  arc A2 (-28.33, 12.83) -> (-27.28, 11.78) centre (-27.28, 12.83) ccw
  line L3 (-27.28, 11.78) -> (-26.72, 11.78)
  arc A3 (-26.72, 11.78) -> (-25.67, 12.83) centre (-26.72, 12.83) ccw
extrude "GCT 8.44 x 2.66 throat R1.05" cut sketch "GCT 8.44 x 2.66 throat R1.05 profile" along normal blind 1.92 bodies 36 in component "USB — removable metal faceplate — local 1.80 mm seat"
ref_plane "WorkPlane4" through (73.09, 0, 0) normal (1, 0, 0) x (0, 1, 0) in component "USB — removable metal faceplate — local 1.80 mm seat"
sketch "GCT 9.14 x 3.35 inner lip R1.39 profile" plane through (73.09, 0, 0) normal (1, 0, 0) x (0, 0, -1) in component "USB — removable metal faceplate — local 1.80 mm seat"
  line L0 (-25.325, 12.82) -> (-25.325, 19.18)
  arc A0 (-25.325, 19.18) -> (-26.715, 20.57) centre (-26.715, 19.18) ccw
  line L1 (-26.715, 20.57) -> (-27.285, 20.57)
  arc A1 (-27.285, 20.57) -> (-28.675, 19.18) centre (-27.285, 19.18) ccw
  line L2 (-28.675, 19.18) -> (-28.675, 12.82)
  arc A2 (-28.675, 12.82) -> (-27.285, 11.43) centre (-27.285, 12.82) ccw
  line L3 (-27.285, 11.43) -> (-26.715, 11.43)
  arc A3 (-26.715, 11.43) -> (-25.325, 12.82) centre (-26.715, 12.82) ccw
extrude "GCT 9.14 x 3.35 inner lip R1.39" cut sketch "GCT 9.14 x 3.35 inner lip R1.39 profile" along normal blind 0.18 bodies 36 in component "USB — removable metal faceplate — local 1.80 mm seat"